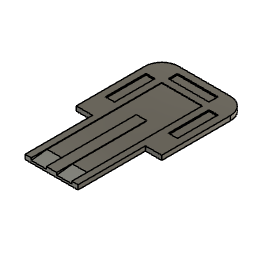
biosensorBottom v2 (Autodesk Fusion 360 design; units mm, degrees)
Autodesk Fusion 360 part; units mm, degrees
sketch "Sketch1" plane through (0, 0, 0) normal (0, 0, 1) x (1, 0, 0)
  line L0 (0, 0) -> (18, 0)
  line L1 (18, 0) -> (18, 18)
  line L2 (18, 18) -> (0, 18)
  line L3 (0, 18) -> (0, 0)
  line L4 (0, 18) -> (-10, 18)
  line L5 (-10, 18) -> (-10, 28)
  line L6 (-10, 28) -> (28, 28)
  line L7 (28, 28) -> (28, -10)
  line L8 (28, -10) -> (-10, -10)
  line L9 (-10, -10) -> (-10, 28)
  dimension "d1" = 18
  dimension "d2" = 18
  dimension "d3" = 10
  dimension "d4" = 10
  dimension "d5" = 10
  dimension "d6" = 10
  constraint horizontal L0
  constraint vertical L1
  constraint horizontal L2
  constraint vertical L3
  constraint coincident L0.start L3.end
  constraint perpendicular L3 L4
  constraint perpendicular L4 L5
  constraint horizontal L6
  constraint vertical L7
  constraint horizontal L8
  constraint vertical L9
  measures "d1" distance of L0.start L0.end
  measures "d2" distance of L0.start L2.end
  measures "d3" distance of L2.end L4.end
  measures "d4" distance of L4.end L5.end
  measures "d5" distance of L1 L7
  measures "d6" distance of L0 L8
extrude "Extrude1" add sketch "Sketch1" along normal blind 2
extrude "Extrude2" add sketch "Sketch1" along normal blind 1.8 contours L0 L1 L2 L3
sketch "Sketch2" plane through (0, -10, 0) normal (0, -1, 0) x (1, 0, 0)
  line L0 (-10, 0) -> (28, 0)
  line L1 (28, 0) -> (28, 2)
  line L2 (28, 2) -> (-10, 2)
  line L3 (-10, 2) -> (-10, 0)
  line L4 (9, 2) -> (-2.75, 2)
  line L5 (9, 2) -> (20.75, 2)
  line L6 (-2.75, 2) -> (-2.75, 0)
  line L7 (20.75, 2) -> (20.75, 0)
  dimension "d11" = 11.75
  dimension "d12" = 11.75
  constraint midpoint L2 L4.start
  constraint parallel L2 L4
  constraint parallel L2 L5
  constraint coincident L0 L6.end
  constraint perpendicular L0 L6
  constraint coincident L0 L7.end
  constraint perpendicular L0 L7
  measures "d11" distance of L4.start L4.end
  measures "d12" distance of L4.start L5.end
extrude "Extrude3" add sketch "Sketch2" along normal blind 30 contours L0 L2 L4 L5 L6 L7
sketch "Sketch3" plane through (0, 0, 2) normal (0, 0, 1) x (-1, 0, 0)
  line L0 (0, 0) -> (0, -18)
  line L1 (0, -18) -> (-18, -18)
  line L2 (-18, -18) -> (-18, 0)
  line L3 (-18, 0) -> (0, 0)
  line L4 (10, 10) -> (2.75, 10)
  line L5 (2.75, 10) -> (2.75, 40)
  line L6 (2.75, 40) -> (-20.75, 40)
  line L7 (-20.75, 40) -> (-20.75, 10)
  line L8 (-20.75, 10) -> (-28, 10)
  line L9 (-28, 10) -> (-28, -28)
  line L10 (-28, -28) -> (10, -28)
  line L11 (10, -28) -> (10, 10)
  line L12 (-9, 40) -> (-9, 0)
  line L13 (-31.221, 25) -> (-24.871, 25)
  line L14 (-9, 40) -> (-20.75, 40)
  line L15 (-9, 40) -> (2.75, 40)
  line L16 (0, 0) -> (0, 40)
  line L17 (0, 40) -> (-6.7, 40)
  line L18 (-6.7, 40) -> (-6.7, 0)
  line L19 (-18, 0) -> (-18, 40)
  line L20 (-11.3, 40) -> (-11.3, 0)
  line L21 (-18, 40) -> (-11.3, 40)
  dimension "d15" = 6.35
  dimension "d18" = 6.7
  constraint midpoint L6 L12.start
  constraint midpoint L3 L12.end
  constraint perpendicular L7 L13
  constraint coincident L6.end L7.start
  constraint coincident L5.end L6.start
  constraint vertical L16
  constraint coincident L0.start L3.end
  constraint coincident L6 L16.end
  constraint coincident L15 L17.end
  constraint coincident L3 L18.end
  constraint perpendicular L3 L18
  constraint symmetric L12 L0.start L2.end
  constraint symmetric L12 L16.end L19.end
  constraint symmetric L12 L17.end L20.start
  constraint symmetric L12 L18.end L20.end
  measures "d15" distance of L13.start L13.end
  measures "d18" distance of L16.end L17.end
extrude "Extrude4" cut sketch "Sketch3" against normal blind 0.2 contours L3 L6 L15 L16 L17 L18 | L3 L6 L14 L19 L20 L21
chamfer "Chamfer1" distance 0.8 distance2 7 2 edges at (14.65, -40, 1.8) (3.35, -40, 1.8) measured on face at (8.2333, -40, 0.6) measured on face at (8.2333, -40, 0.6)
fillet "Fillet1" radius 7.5 2 edges at (-10, 28, 1) (28, 28, 1)
sketch "Sketch4" plane through (0, 0, 2) normal (0, 0, 1) x (-1, 0, 0)
  arc A0 (-28, -20.5) -> (-20.5, -28) centre (-20.5, -20.5) ccw
  line L0 (-20.5, -28) -> (2.5, -28)
  arc A1 (2.5, -28) -> (10, -20.5) centre (2.5, -20.5) ccw
  line L1 (10, -20.5) -> (10, 10)
  line L2 (10, 10) -> (2.75, 10)
  line L3 (2.75, 10) -> (2.75, 40)
  line L4 (2.75, 40) -> (0, 40)
  line L5 (0, 40) -> (0, -18)
  line L6 (0, -18) -> (-18, -18)
  line L7 (-18, -18) -> (-18, 40)
  line L8 (-18, 40) -> (-20.75, 40)
  line L9 (-20.75, 40) -> (-20.75, 10)
  line L10 (-20.75, 10) -> (-28, 10)
  line L11 (-28, 10) -> (-28, -20.5)
  line L12 (0, -18) -> (10, -18)
  line L13 (5, -18) -> (5, 0)
  line L14 (5, 0) -> (3, 0)
  line L15 (3, 0) -> (3, -18)
  line L16 (5, 0) -> (7, 0)
  line L17 (7, 0) -> (7, -18)
  line L18 (-9, -18) -> (-9, -9)
  line L19 (-25, 0) -> (-25, -18)
  line L20 (-23, -18) -> (-23, 0)
  line L21 (-21, 0) -> (-21, -18)
  line L22 (-18, -18) -> (-28, -18)
  line L23 (-23, 0) -> (-21, 0)
  line L24 (-23, 0) -> (-25, 0)
  line L25 (-18, -18) -> (0, 0)
  line L26 (0, -21) -> (-18, -21)
  line L27 (-18, -23) -> (0, -23)
  line L28 (0, -25) -> (-18, -25)
  line L29 (-18, -18) -> (-18, -28)
  line L30 (0, -23) -> (0, -21)
  line L31 (0, -23) -> (0, -25)
  dimension "d25" = 2
  dimension "d26" = 2
  constraint coincident L5.end L6.start
  constraint coincident L1 L12.end
  constraint perpendicular L1 L12
  constraint midpoint L12 L13.start
  constraint perpendicular L2 L13
  constraint perpendicular L13 L14
  constraint perpendicular L14 L15
  constraint perpendicular L13 L16
  constraint coincident L12 L17.end
  constraint perpendicular L12 L17
  constraint midpoint L6 L18.start
  constraint perpendicular L6 L18
  constraint symmetric L5.end L18 L6.end
  constraint symmetric L12.end L18 L22.end
  constraint symmetric L13.start L18 L20.start
  constraint symmetric L13.end L18 L20.end
  constraint symmetric L14.end L18 L21.start
  constraint symmetric L15.end L18 L21.end
  constraint symmetric L16.end L18 L19.start
  constraint symmetric L17.end L18 L19.end
  constraint coincident L6.end L7.start
  constraint coincident L25.end origin
  constraint symmetric L19.start L25 L28.start
  constraint symmetric L19.end L25 L28.end
  constraint symmetric L20.start L25 L27.start
  constraint symmetric L20.end L25 L27.end
  constraint symmetric L21.start L25 L26.start
  constraint symmetric L21.end L25 L26.end
  constraint symmetric L6.end L25 L7.start
  constraint symmetric L22.end L25 L29.end
  measures "d25" distance of L13.end L14.end
  measures "d26" distance of L13.end L16.end
extrude "Extrude5" cut sketch "Sketch4" against normal blind 0.6 contours L19 L20 L22 L24 | L27 L28 L29 L31 | L20 L21 L22 L23 | L26 L27 L29 L30 | L12 L13 L16 L17 | L12 L13 L14 L15
